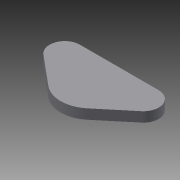
# Autodesk Inventor part: body-back
Saved by Autodesk Inventor 2013 (Build 170138000, 138)
## iProperties
Created: 2012-09-08
Part Number: body-back
Material: Generic
Document SubType Name: Modeling
Designer: frankenteddy
Density: 1 g/cm^3
Author: frankenteddy
Autodesk Inventor part; units mm, degrees
ref_plane "YZ Plane" through (0, 0, 0) normal (1, 0, 0) x (0, 1, 0)
ref_plane "XZ Plane" through (0, 0, 0) normal (0, 1, 0) x (-1, 0, 0)
ref_plane "XY Plane" through (0, 0, 0) normal (0, 0, 1) x (1, 0, 0)
sketch "Sketch1" plane through (0, 0, 0) normal (0, 0, 1) x (1, 0, 0)
  line L0 (-92.7646, -8.503) -> (-89.7646, -8.503)
  line L1 (-89.7646, -8.503) -> (-89.7646, -11.753)
  line L2 (-89.7646, -11.753) -> (-92.7646, -11.753)
  line L3 (-92.7646, -11.753) -> (-92.7646, -8.503)
  line L4 (-92.7646, -21.6527) -> (-89.7646, -21.6527)
  line L5 (-89.7646, -21.6527) -> (-89.7646, -21.7527)
  line L6 (-89.7646, -21.7527) -> (-92.7646, -21.7527)
  line L7 (-92.7646, -21.7527) -> (-92.7646, -21.6527)
  line L8 (-43.5121, 19.6165) -> (76.4879, 19.6165)
  line L9 (76.4879, 19.6165) -> (76.4879, 99.6165)
  line L10 (76.4879, 99.6165) -> (-43.5121, 99.6165)
  line L11 (-43.5121, 99.6165) -> (-43.5121, 19.6165)
  line L12 (16.4879, 99.6165) -> (16.4879, 19.6165) construction
  line L13 (-43.5121, 59.6165) -> (76.4879, 59.6165) construction
  line L14 (3.9879, 63.1165) -> (7.2379, 63.1165)
  line L15 (7.2379, 63.1165) -> (7.2379, 56.1165)
  line L16 (7.2379, 56.1165) -> (3.9879, 56.1165)
  line L17 (3.9879, 56.1165) -> (3.9879, 63.1165)
  line L18 (3.9879, 59.6165) -> (7.2379, 59.6165) construction
  line L19 (28.9879, 63.1165) -> (25.7379, 63.1165)
  line L20 (25.7379, 63.1165) -> (25.7379, 56.1165)
  line L21 (25.7379, 56.1165) -> (28.9879, 56.1165)
  line L22 (28.9879, 56.1165) -> (28.9879, 63.1165)
  line L23 (28.9879, 59.6165) -> (25.7379, 59.6165) construction
  circle A0 centre (-1.5121, 74.6165) radius 5
  circle A1 centre (34.4879, 74.6165) radius 5
  circle A2 centre (-3.5121, 37.1165) radius 2.5
  circle A3 centre (6.4879, 37.1165) radius 2.5
  circle A4 centre (16.4879, 37.1165) radius 2.5
  circle A5 centre (26.4879, 37.1165) radius 2.5
  circle A6 centre (36.4879, 37.1165) radius 2.5
  circle A7 centre (-3.5121, 44.1165) radius 2.5
  line L24 (-6.0121, 37.1165) -> (-1.0121, 37.1165) construction
  circle A8 centre (-3.5121, 30.1165) radius 2.5
  line L25 (6.4879, 39.6165) -> (6.4879, 34.6165) construction
  circle A9 centre (36.4879, 44.1165) radius 2.5
  circle A10 centre (36.4879, 30.1165) radius 2.5
  circle A11 centre (16.4879, 30.1165) radius 2.5
  line L26 (-43.5121, 99.6165) -> (-53.5121, 99.6165)
  line L27 (-53.5121, 99.6165) -> (-53.5121, 19.6165)
  line L28 (-53.5121, 19.6165) -> (-43.5121, 19.6165)
  line L29 (-43.5121, 19.6165) -> (-43.5121, 99.6165)
  arc A12 (16.4879, 99.6165) -> (-34.1013, 83.0147) centre (13.3048, 23.9368) ccw
  arc A13 (-34.1013, 36.2182) -> (16.4879, 19.6165) centre (13.3048, 95.2961) ccw
  arc A14 (-34.1013, 83.0147) -> (-34.1013, 36.2182) centre (-15.3258, 59.6165) ccw
  arc A15 (67.0771, 83.0147) -> (16.4879, 99.6165) centre (19.6709, 23.9368) ccw
  arc A16 (16.4879, 19.6165) -> (67.0771, 36.2182) centre (19.6709, 95.2961) ccw
  arc A17 (67.0771, 36.2182) -> (67.0771, 83.0147) centre (48.3015, 59.6165) ccw
  line L30 (10.086, 48.1846) -> (0.2957, 56.3433)
  line L31 (3.4966, 65.1844) -> (16.4879, 65.1844)
  arc A18 (3.4966, 65.1844) -> (0.2957, 56.3433) centre (3.4966, 60.1844) ccw
  line L32 (22.8898, 48.1846) -> (32.6801, 56.3433)
  line L33 (29.4791, 65.1844) -> (16.4879, 65.1844)
  arc A19 (32.6801, 56.3433) -> (29.4791, 65.1844) centre (29.4791, 60.1844) ccw
  arc A20 (10.086, 48.1846) -> (22.8898, 48.1846) centre (16.4879, 55.8667) ccw
  point P0 (0, 0)
  point P1 (16.4879, 42.8496)
  dimension "d3" = 3
  dimension "mat" = 3.25
  dimension "d5" = 3
  dimension "kerf" = 0.1
  dimension "d42" = 120
  dimension "d43" = 80
  dimension "d44" = 3.25
  dimension "d45" = 7
  dimension "d47" = 9.25
  dimension "d50" = 10
  dimension "d51" = 13
  dimension "d54" = 20
  dimension "d55" = 5
  dimension "d58" = 10
  dimension "d63" = 15
  dimension "d64" = 5
  dimension "d65" = 7
  dimension "d69" = 10
  dimension "d70" = 30
  dimension "d73" = 5
  dimension "d74" = 10
  constraints: 68 end point, 22 point on circle, 21 centre point, 20 symmetric about line, 10 parallel, 8 perpendicular, 6 horizontal, 6 midpoint, 6 tangent, 5 point on line, 1 collinear, 18 other
  measures "d3" distance of L1.end L2.end
  measures "mat" distance of L0.end L1.end
  measures "d5" distance of L5.end L6.end
  measures "kerf" distance of L4.end L5.end
  measures "d42" distance of L10.end L9.end
  measures "d43" distance of L9.end L8.end
  measures "d44" distance of L15.end L16.end
  measures "d45" distance of L14.end L15.end
  measures "d47" distance between parallel lines of L12 L15
  measures "d50" diameter of A0
  measures "d51" distance edge to line of A0 L12
  measures "d54" distance edge to line of A0 L10
  measures "d55" diameter of A2
  measures "d58" distance of A2.centre A3.centre
  measures "d63" distance edge to line of A4 L8
  measures "d64" diameter of A7
  measures "d65" distance of A2.centre A7.centre
  measures "d69" distance of L28.end L27.end
  measures "d70" radius of A14
  measures "d73" radius of A18
  measures "d74" radius of A20
extrude "Extrusion11" add sketch "Sketch1" along normal blind 3.25 contours L14 L15 L16 L17 | L22 L21 L20 L19 | L30 A18 L31 L33 A19 L32 A20
equation "\"d44\" = mat"
equation "\"d77\" = mat"
body "Solid5"
